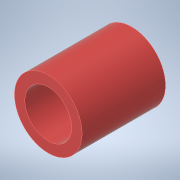
# Autodesk Inventor part: Spacer Creator
Saved by Autodesk Inventor 2022.3 (Build 263350000, 350)
## iProperties
Created: 2023-02-19
Part Number: Spacer Creator
Material: ABS Plastic
Document SubType Name: Modeling
Designer: mavericks
Density: 1.06 g/cm^3
Appearance: Smooth - Red
RuleStatus: InUse
AfterDocNew0: Open Form 1
Author: mavericks
Autodesk Inventor part; units mm, degrees
ref_plane "YZ Plane" through (0, 0, 0) normal (1, 0, 0) x (0, 1, 0)
ref_plane "XZ Plane" through (0, 0, 0) normal (0, 1, 0) x (-1, 0, 0)
ref_plane "XY Plane" through (0, 0, 0) normal (0, 0, 1) x (1, 0, 0)
sketch "Sketch1" plane through (0, 0, 0) normal (0, 0, 1) x (1, 0, 0)
  circle A0 centre (0, 0) radius 7.125
  circle A1 centre (0, 0) radius 10.3
  dimension "d13" = 14.25
  dimension "d14" = 3.175
  constraints: 2 centre point, 1 coincident, 1 other
  measures "d13" diameter of A0
  measures "d14" radial gap between concentric circles of A0 A1
extrude "Extrusion1" add sketch "Sketch1" along normal blind 25.4
equation "\"d13\" = HoleDiameter"
equation "\"d1\" = SpacerLength"
equation "\"SpacerLength\" = 25.4"
equation "\"HoleDiameter\" = 14.25"
body "Solid1"
